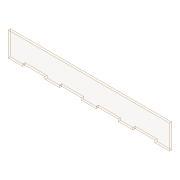
# Autodesk Inventor part: Divisória-22cm
Saved by Autodesk Inventor 2020 (Build 240168000, 168)
## iProperties
Created: 2021-09-21
Part Number: Divisória-22cm
Material: Generic
Document SubType Name: Modeling
Designer: pablo
Density: 1 g/cm^3
Appearance: Polycarbonate - Smoked
Author: pablo
Autodesk Inventor part; units mm, degrees
ref_plane "YZ Plane" through (0, 0, 0) normal (1, 0, 0) x (0, 1, 0)
ref_plane "XZ Plane" through (0, 0, 0) normal (0, 1, 0) x (-1, 0, 0)
ref_plane "XY Plane" through (0, 0, 0) normal (0, 0, 1) x (1, 0, 0)
sketch "Sketch1" plane through (0, 0, 0) normal (0, 0, 1) x (1, 0, 0)
  line L0 (-110, 15) -> (110, 15)
  line L1 (110, 15) -> (110, -15)
  line L2 (110, -15) -> (-110, -15)
  line L3 (-110, -15) -> (-110, 15)
  line L4 (-110, 15) -> (110, -15) construction
  line L5 (110, 15) -> (-110, -15) construction
  point P0 (0, 0)
  dimension "d0" = 220
  dimension "d1" = 30
  constraints: 12 end point, 2 midpoint, 2 parallel, 1 horizontal, 1 perpendicular
  measures "d0" distance of L1.end L2.end
  measures "d1" distance of L0.end L1.end
extrude "Base" add sketch "Sketch1" along normal blind 3
sketch "Sketch2" plane through (0, 0, 3) normal (0, 0, 1) x (1, 0, 0)
  line L0 (-110, -15) -> (110, -15) projected
  line L1 (-110, -15) -> (-90, -15)
  line L2 (-90, -15) -> (-90, -18)
  line L3 (-90, -18) -> (-110, -18)
  line L4 (-110, -18) -> (-110, -15)
  line L5 (-60, -15) -> (-40, -15)
  line L6 (-40, -15) -> (-40, -18)
  line L7 (-40, -18) -> (-60, -18)
  line L8 (-60, -18) -> (-60, -15)
  line L9 (-10, -15) -> (10, -15)
  line L10 (10, -15) -> (10, -18)
  line L11 (10, -18) -> (-10, -18)
  line L12 (-10, -18) -> (-10, -15)
  line L13 (40, -15) -> (60, -15)
  line L14 (60, -15) -> (60, -18)
  line L15 (60, -18) -> (40, -18)
  line L16 (40, -18) -> (40, -15)
  line L17 (90, -15) -> (110, -15)
  line L18 (110, -15) -> (110, -18)
  line L19 (110, -18) -> (90, -18)
  line L20 (90, -18) -> (90, -15)
  point P0 (0, 0)
  point P1 (60, -15)
  point P2 (10, -15)
  point P3 (-90, -15)
  point P4 (90, -15)
  point P5 (-40, -15)
  dimension "d4" = 20
  dimension "d5" = 3
  dimension "d8" = 50
  constraints: 40 end point, 2 horizontal, 2 parallel, 1 perpendicular, 32 other
  measures "d4" distance of L2.end L3.end
  measures "d5" distance of L1.end L2.end
  measures "d8" distance of L2.end L6.end
extrude "Encaixe" add sketch "Sketch2" against normal blind 3
body "Solid1"
